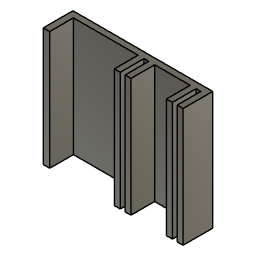
Shelf supports (Autodesk Fusion 360 design; units mm, degrees)
Autodesk Fusion 360 part; units mm, degrees
sketch "Sketch6" plane through (0, 0, 0) normal (0, 0, 1) x (1, 0, 0)
  line L0 (59, -2.5) -> (-59, -2.5)
  line L1 (-59, -2.5) -> (-59, 2.5)
  line L2 (-59, 2.5) -> (59, 2.5)
  line L3 (59, 2.5) -> (59, -2.5)
  line L4 (59, -2.5) -> (-59, 2.5) construction
  line L5 (-59, -2.5) -> (59, 2.5) construction
  dimension "d8" = 118
  dimension "d9" = 5
  constraint horizontal L0
  constraint perpendicular L0 L1
  constraint parallel L0 L2
  constraint parallel L1 L3
  constraint coincident L4 origin
  constraint coincident L5 origin
  measures "d8" distance of L1 L3
  measures "d9" distance of L0 L2
sketch "Sketch7" plane through (0, 0, 0) normal (0, 0, 1) x (1, 0, 0)
  line L0 (-464, -2.5) -> (-459, -2.5)
  line L1 (-459, -2.5) -> (-459, -22.5)
  line L2 (-459, -22.5) -> (-464, -22.5)
  line L3 (-464, -22.5) -> (-464, -2.5)
  line L4 (-459, -22.5) -> (-464, -22.5)
  line L5 (-464, -22.5) -> (-464, -2.5)
  line L6 (-459, -2.5) -> (-459, -22.5)
  line L7 (-464, -2.5) -> (-459, -2.5)
  dimension "d10" = 5
  dimension "d11" = 20
  dimension "d12" = 5
  dimension "d13" = 20
  constraint horizontal L0
  constraint vertical L1
  constraint horizontal L2
  constraint vertical L3
  constraint horizontal L7
  constraint vertical L6
  constraint horizontal L4
  constraint vertical L5
  measures "d10" distance of L1 L3
  measures "d11" distance of L0 L2
  measures "d12" distance of L5 L6
  measures "d13" distance of L4 L7
sketch "Sketch8" plane through (0, 0, 0) normal (0, 0, 1) x (1, 0, 0)
  line L0 (136, -2.5) -> (141, -2.5)
  line L1 (141, -2.5) -> (141, -22.5)
  line L2 (141, -22.5) -> (136, -22.5)
  line L3 (136, -22.5) -> (136, -2.5)
  dimension "d14" = 5
  dimension "d15" = 20
  constraint horizontal L0
  constraint vertical L1
  constraint horizontal L2
  constraint vertical L3
  measures "d14" distance of L1 L3
  measures "d15" distance of L0 L2
sketch "Sketch9" plane through (0, 0, 0) normal (0, 0, 1) x (1, 0, 0)
  line L0 (459, -2.5) -> (464, -2.5)
  line L1 (464, -2.5) -> (464, -22.5)
  line L2 (464, -22.5) -> (459, -22.5)
  line L3 (459, -22.5) -> (459, -2.5)
  dimension "d16" = 5
  dimension "d17" = 20
  constraint horizontal L0
  constraint vertical L1
  constraint horizontal L2
  constraint vertical L3
  measures "d16" distance of L1 L3
  measures "d17" distance of L0 L2
sketch "Sketch10" plane through (0, 0, 0) normal (0, 0, 1) x (1, 0, 0)
  line L0 (450, -2.5) -> (455, -2.5)
  line L1 (455, -2.5) -> (455, -22.5)
  line L2 (455, -22.5) -> (450, -22.5)
  line L3 (450, -22.5) -> (450, -2.5)
  dimension "d20" = 5
  dimension "d21" = 20
  constraint horizontal L0
  constraint vertical L1
  constraint horizontal L2
  constraint vertical L3
  measures "d20" distance of L1 L3
  measures "d21" distance of L0 L2
sketch "Sketch11" plane through (0, 0, 0) normal (0, 0, 1) x (1, 0, 0)
  line L0 (145, -2.5) -> (150, -2.5)
  line L1 (150, -2.5) -> (150, -22.5)
  line L2 (150, -22.5) -> (145, -22.5)
  line L3 (145, -22.5) -> (145, -2.5)
  dimension "d22" = 5
  dimension "d23" = 20
  constraint horizontal L0
  constraint vertical L1
  constraint horizontal L2
  constraint vertical L3
  measures "d22" distance of L1 L3
  measures "d23" distance of L0 L2
extrude "Extrude1" add sketch "Sketch6" along normal blind 100 makes body 1
extrude "Extrude2" add sketch "Sketch7" along normal blind 100 bodies 1 makes body 2
extrude "Extrude3" add sketch "Sketch8" along normal blind 100 bodies 2 1 makes body 3
extrude "Extrude4" add sketch "Sketch11" along normal blind 100 bodies 3 2 1 makes body 4
extrude "Extrude5" add sketch "Sketch10" along normal blind 100 bodies 4 3 2 1 makes body 5
extrude "Extrude6" add sketch "Sketch9" along normal blind 100 bodies 5 4 3 2 1 makes body 6
move_body "Move1" bodies 2 to x (1, 0, 0) y (0, 1, 0) z (0, 0, 1) at (418, 0, 0)
move_face "MoveFace1" by (-0.4, 0, 0) 1 faces at (-46, -15.8333, 33.3333) on bodies 2
move_body "Move2" bodies 5 6 to x (1, 0, 0) y (0, 1, 0) z (0, 0, 1) at (-417.6, 0, 0)
move_body "Move3" bodies 4 3 to x (1, 0, 0) y (0, 1, 0) z (0, 0, 1) at (-140, 0, 0)
move_body "Move4" bodies 3 4 to x (1, 0, 0) y (0, 1, 0) z (0, 0, 1) at (5, 0, 0)
move_body "Move5" bodies 4 3 to x (1, 0, 0) y (0, 1, 0) z (0, 0, 1) at (7, 0, 0)
move_body "Move6" bodies 4 3 to x (1, 0, 0) y (0, 1, 0) z (0, 0, 1) at (4, 0, 0)
move_body "Move7" bodies 2 to x (1, 0, 0) y (0, 1, 0) z (0, 0, 1) at (-12.6, 0, 0)
move_body "Move8" bodies 6 5 to x (1, 0, 0) y (0, 1, 0) z (0, 0, 1) at (12.6, 0, 0)
move_body "Move9" bodies 4 3 to x (1, 0, 0) y (0, 1, 0) z (0, 0, 1) at (-11, 0, 0)
combine "Combine1" operation add target body 1 tool bodies 2 3 4 6 5
